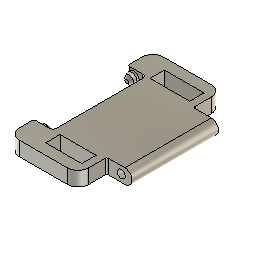
Cadena Oruga (Autodesk Fusion 360 archive; units mm, degrees)
design "Eslabón"
Autodesk Fusion 360 part; units mm, degrees
sketch "Boceto1" plane through (0, 0, 0) normal (0, 0, 1) x (1, 0, 0)
  line L0 (0, 0) -> (15, 0)
  line L1 (15, 0) -> (15, 30)
  line L2 (15, 30) -> (0, 30)
  line L3 (0, 28) -> (0, 2)
  line L4 (0, 30) -> (-7, 30)
  line L5 (-7, 30) -> (-7, 28)
  line L6 (-7, 28) -> (0, 28)
  line L7 (0, 0) -> (-7, 0)
  line L8 (-7, 0) -> (-7, 2)
  line L9 (-7, 2) -> (0, 2)
  line L10 (15, 30) -> (15, 27)
  line L11 (15, 27) -> (21, 27)
  line L12 (15, 24) -> (15, 27)
  line L13 (15, 0) -> (15, 3)
  line L14 (15, 3) -> (21, 3)
  line L15 (15, 6) -> (15, 3)
  line L16 (15, 6) -> (15, 24)
  line L17 (21, 27) -> (21, 3)
  dimension "d1" = 15
  dimension "d3" = 3
  dimension "d4" = 3
  dimension "d14" = 7
  dimension "d15" = 7
  dimension "d16" = 6
  constraint horizontal L0
  constraint vertical L1
  constraint horizontal L2
  constraint vertical L3
  constraint coincident L0.start L7.start
  constraint horizontal L4
  constraint vertical L5
  constraint horizontal L6
  constraint horizontal L7
  constraint vertical L8
  constraint horizontal L9
  constraint coincident L1 L10.end
  constraint horizontal L11
  constraint vertical L12
  constraint coincident L1 L13.end
  constraint horizontal L14
  constraint vertical L15
  constraint vertical L16
  constraint perpendicular L14 L17
  measures "d1" distance of L0.start L0.end
  measures "d3" distance of L1.end L10.end
  measures "d4" distance of L0.end L13.end
  measures "d14" distance of L2.end L4.end
  measures "d15" distance of L0.start L7.end
  measures "d16" distance of L10.end L11.end
extrude "Extruir1" add sketch "Boceto1" along normal blind 4 makes body 1
sketch "Boceto2" plane through (0, 28, 0) normal (0, -1, 0) x (1, 0, 0)
  line L0 (-7, 0) -> (0, 0)
  line L1 (0, 0) -> (0, 4)
  line L2 (0, 4) -> (-7, 4)
  line L3 (-7, 4) -> (-7, 0)
  line L4 (0, 4) -> (-3.5, 4)
  line L5 (-3.5, 4) -> (-3.5, 2)
  circle A0 centre (-3.5, 2) radius 1.5
  constraint coincident L1.end L2.start
  constraint midpoint L2 L4.end
  constraint perpendicular L0 L5
  constraint coincident L5.end A0.centre
extrude "Extruir2" add sketch "Boceto2" along normal blind 2 contours A0 bodies 1
chamfer "Chaflán1" distance 1 angle 45 1 edges at (-4.8985, 26, 1.4576) on bodies 1
sketch "Boceto3" plane through (0, 2, 0) normal (0, 1, 0) x (-1, 0, 0)
  line L0 (0, 0) -> (7, 0)
  line L1 (7, 0) -> (7, 4)
  line L2 (7, 4) -> (0, 4)
  line L3 (0, 4) -> (0, 0)
  line L4 (3.5, 4) -> (3.5, 2)
  circle A0 centre (3.5, 2) radius 1.5
  dimension "d21" = 3
  constraint midpoint L2 L4.start
  constraint perpendicular L2 L4
  constraint coincident L4.end A0.centre
  measures "d21" diameter of A0
extrude "Extruir3" add sketch "Boceto3" along normal blind 2 contours A0 bodies 1
chamfer "Chaflán2" distance 1 angle 45 1 edges at (-2.1015, 4, 1.4576) on bodies 1
move_face "CarasDesfase1" offset 5 2 faces at (7.6667, 0, 1.3333) (7.6667, 30, 1.3333) on bodies 1
sketch "Boceto4" plane through (0, 3, 0) normal (0, -1, 0) x (1, 0, 0)
  line L0 (15, 0) -> (21, 0)
  line L1 (21, 0) -> (21, 4)
  line L2 (21, 4) -> (15, 4)
  line L3 (15, 4) -> (15, 0)
  line L4 (18, 4) -> (18, 2)
  circle A0 centre (18, 2) radius 1.5
  dimension "d20" = 3
  constraint midpoint L2 L4.start
  constraint perpendicular L2 L4
  constraint coincident L4.end A0.centre
  measures "d20" diameter of A0
extrude "Extruir4" cut sketch "Boceto4" against normal blind 2 contours A0 bodies 1
sketch "Boceto5" plane through (0, 27, 0) normal (0, 1, 0) x (-1, 0, 0)
  line L0 (-21, 0) -> (-15, 0)
  line L1 (-15, 0) -> (-15, 4)
  line L2 (-15, 4) -> (-21, 4)
  line L3 (-21, 4) -> (-21, 0)
  line L4 (-18, 4) -> (-18, 2)
  circle A0 centre (-18, 2) radius 1.5
  dimension "d24" = 3
  constraint midpoint L2 L4.start
  constraint perpendicular L2 L4
  constraint coincident L4.end A0.centre
  measures "d24" diameter of A0
extrude "Extruir5" cut sketch "Boceto5" against normal blind 2 contours A0 bodies 1
copy_body "Cuerpo - > Comp.1" bodies 1 removing the originals makes body 2 in component "Eslabón"
sketch "Boceto6" plane through (0, 0, 4) normal (0, 0, 1) x (-1, 0, 0)
  line L0 (-15, 5) -> (-15, -3)
  line L1 (-15, -3) -> (-21, -3)
  line L2 (-21, -3) -> (-21, -27)
  line L3 (-21, -27) -> (-15, -27)
  line L4 (-15, -27) -> (-15, -35)
  line L5 (-15, -35) -> (7, -35)
  line L6 (7, -35) -> (7, -28)
  line L7 (7, -28) -> (0, -28)
  line L8 (0, -28) -> (0, -2)
  line L9 (0, -2) -> (7, -2)
  line L10 (7, -2) -> (7, 5)
  line L11 (7, 5) -> (-15, 5)
  line L12 (0, -2) -> (-1, -2)
  line L13 (-2, -2) -> (-12, -2)
  line L14 (-12, -2) -> (-12, 2)
  line L15 (-12, 2) -> (-2, 2)
  line L16 (-2, 2) -> (-2, -2)
  line L17 (0, -28) -> (-1, -28)
  line L18 (-1, -28) -> (-12, -28)
  line L19 (-12, -28) -> (-12, -32)
  line L20 (-12, -32) -> (-1, -32)
  line L21 (-1, -32) -> (-1, -28)
  dimension "d49" = 1
  dimension "d50" = 1
  constraint coincident L8.end L9.start
  constraint perpendicular L8 L12
  constraint horizontal L13
  constraint vertical L14
  constraint horizontal L15
  constraint vertical L16
  constraint coincident L12 L13.start
  constraint coincident L7.end L8.start
  constraint perpendicular L8 L17
  constraint horizontal L18
  constraint vertical L19
  constraint horizontal L20
  constraint vertical L21
  measures "d49" distance of L7.end L17.end
  measures "d50" distance of L8.end L12.end
extrude "Extruir1'" cut sketch "Boceto6" against normal blind 6 contours L13 L14 L15 L16 | L18 L19 L20 L21 bodies 2 in component "Eslabón"
fillet "Empalme1" radius 1 2 edges at (0, 28, 2) (0, 2, 2) on bodies 2 in component "Eslabón"
fillet "Empalme2" radius 1 2 edges at (-4.8985, 27, 1.4576) (-2.1015, 3, 1.4576) on bodies 2 in component "Eslabón"
fillet "Empalme3" radius 0.5 2 edges at (15, 3, 2) (15, 27, 2) on bodies 2 in component "Eslabón"
move_face "CarasDesfase1'" offset -1.75 2 faces at (-7, 32.6667, 1.3333) (-7, -2.6667, 1.3333) on bodies 2 in component "Eslabón"
fillet "Empalme4" radius 3 2 edges at (-5.25, 35, 2) (-5.25, -5, 2) on bodies 2 in component "Eslabón"
fillet "Empalme6" radius 0.5 2 edges at (-5.25, 28, 2) (-5.25, 2, 2) on bodies 2 in component "Eslabón"
move_face "CarasDesfase2" offset -1 2 faces at (15, 30, 1.3333) (15, -2.5, 1.3333) on bodies 2 in component "Eslabón"
fillet "Empalme7" radius 3 2 edges at (14, -5, 2) (14, 35, 2) on bodies 2 in component "Eslabón"
fillet "Empalme8" radius 2 2 edges at (21, 15, 4) (21, 15, 0) on bodies 2 in component "Eslabón"
move_face "CarasDesfase3" offset 0.4 1 faces at (19.4925, 4.3333, 1.8506) on bodies 2 in component "Eslabón"
component "Eslabón" placed x (1, 0, 0) y (0, 1, 0) z (0, 0, 1) at (0, 0, 0)
named bodies: "Eslabón"
